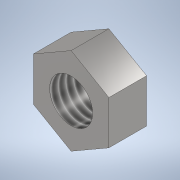
# Autodesk Inventor part: tuercaM4
Saved by Autodesk Inventor 2021.5 (Build 255421000, 421)
## iProperties
Created: 2024-11-29
Part Number: tuercaM4
Material: Acero inoxidable
Document SubType Name: Modeling
Designer: Joho_
Mass: 0.836328 g
Surface Area: 1.88591 cm^2
Volume: 0.104541 cm^3
Density: 8 g/cm^3
Appearance: Semipulido
Author: Joho_
Autodesk Inventor part; units mm, degrees
ref_plane "YZ Plane" through (0, 0, 0) normal (1, 0, 0) x (0, 1, 0)
ref_plane "XZ Plane" through (0, 0, 0) normal (0, 1, 0) x (-1, 0, 0)
ref_plane "XY Plane" through (0, 0, 0) normal (0, 0, 1) x (1, 0, 0)
sketch "Boceto1" plane through (0, 0, 0) normal (0, 0, 1) x (1, 0, 0)
  circle A0 centre (0, 0) radius 2
  line L0 (0, 0) -> (3.5, 0)
  line L1 (3.5, -2.0207) -> (0, -4.0415)
  line L2 (0, -4.0415) -> (-3.5, -2.0207)
  line L3 (-3.5, -2.0207) -> (-3.5, 2.0207)
  line L4 (-3.5, 2.0207) -> (0, 4.0415)
  line L5 (0, 4.0415) -> (3.5, 2.0207)
  line L6 (3.5, 2.0207) -> (3.5, -2.0207)
  dimension "d0" = 4
  dimension "d1" = 3.5
  constraints: 14 end point, 2 coincident, 1 centre point, 1 horizontal, 1 midpoint, 13 other
  measures "d0" diameter of A0
  measures "d1" distance of L0.start L0.end
extrude "Extrusión1" add sketch "Boceto1" along normal mid plane 3.5
thread "Rosca1" size "M4x0.7" class "6H" standard "ANSI Metric M Profile" full length
